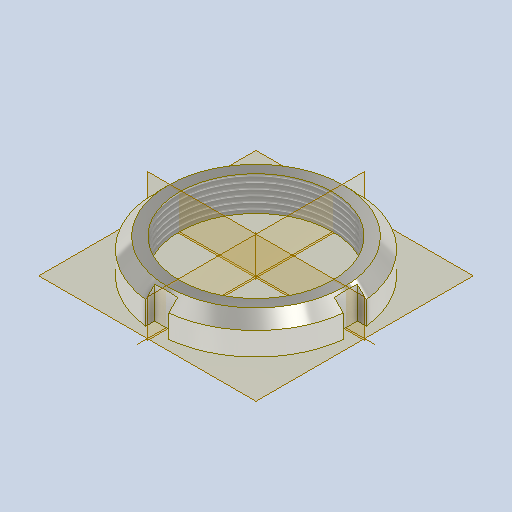
# Autodesk Inventor part: Sicherheitsmutter_m40
Saved by Autodesk Inventor 2022 (Build 260153000, 153)
## iProperties
Created: 2022-03-11
Part Number: Sicherheitsmutter_m40
Material: Generisch
Document SubType Name: Modeling
Designer: 123St
Density: 1 g/cm^3
Appearance: Silber
Mass: 6.67374 g
Surface Area: 40.864 cm^2
Volume: 6.67374 cm^3
Author: 123St
Autodesk Inventor part; units mm, degrees
sketch "Skizze1" plane through (0, 0, 0) normal (0, 1, 0) x (-1, 0, 0)
  circle A0 centre (0, 0) radius 20
  circle A1 centre (0, 0) radius 26
  dimension "d0" = 40
  dimension "d1" = 52
  constraints: 2 centre point, 2 coincident
  measures "d0" diameter of A0
  measures "d1" diameter of A1
extrude "Extrusion1" add sketch "Skizze1" along normal blind 9
chamfer "Fase1" distance 3 angle 45 1 edges at (26, 9, 0)
sketch "Skizze2" plane through (0, 9, 0) normal (0, 1, 0) x (1, 0, 0)
  line L0 (-28.5, -3) -> (-23.5, -3)
  line L1 (-23.5, -3) -> (-23.5, 3)
  line L2 (-23.5, 3) -> (-28.5, 3)
  line L3 (-28.5, 3) -> (-28.5, -3)
  circle A0 centre (0, 0) radius 26 projected
  line L4 (-28.5, -3) -> (-23.5, 3) construction
  line L5 (-23.5, -3) -> (-28.5, 3) construction
  line L6 (3, 23.5) -> (-3, 23.5)
  line L7 (-3, 23.5) -> (-3, 28.5)
  line L8 (-3, 28.5) -> (3, 28.5)
  line L9 (3, 28.5) -> (3, 23.5)
  line L10 (3, 23.5) -> (-3, 28.5) construction
  line L11 (-3, 23.5) -> (3, 28.5) construction
  line L12 (3, -23.5) -> (-3, -23.5)
  line L13 (-3, -23.5) -> (-3, -28.5)
  line L14 (-3, -28.5) -> (3, -28.5)
  line L15 (3, -28.5) -> (3, -23.5)
  line L16 (3, -23.5) -> (-3, -28.5) construction
  line L17 (-3, -23.5) -> (3, -28.5) construction
  line L18 (23.5, -3) -> (28.5, -3)
  line L19 (28.5, -3) -> (28.5, 3)
  line L20 (28.5, 3) -> (23.5, 3)
  line L21 (23.5, 3) -> (23.5, -3)
  line L22 (23.5, -3) -> (28.5, 3) construction
  line L23 (28.5, -3) -> (23.5, 3) construction
  line L24 (-39.9, 0) -> (39.9, 0) projected
  point P0 (-26, 0)
  point P1 (0, 26)
  point P2 (0, -26)
  point P3 (26, 0)
  dimension "d7" = 5
  dimension "d8" = 6
  dimension "d9" = 5
  dimension "d10" = 26
  dimension "d11" = 6
  dimension "d12" = 0
  dimension "d13" = 6
  dimension "d14" = 5
  dimension "d15" = 5
  dimension "d16" = 0
  constraints: 48 end point, 8 midpoint, 8 parallel, 4 horizontal, 4 perpendicular, 3 point on circle, 1 point on line
  measures "d7" distance of L6.end L7.end
  measures "d8" distance of L7.end L8.end
  measures "d9" distance of L19.end L20.end
  measures "d10" distance of A0.centre point (26, 0)
  measures "d11" distance of L18.end L19.end
  measures "d12" distance from line of L24 point (26, 0)
  measures "d13" distance of L13.end L14.end
  measures "d14" distance of L14.end L12.start
  measures "d15" distance of L1.end L2.end
  measures "d16" distance from line of L24 A0.start
extrude "Extrusion2" cut sketch "Skizze2" against normal blind 9 contours L3 L24 A0 L0 | A0 L24 L1 L0 | L3 L2 A0 L24 | A0 L2 L1 L24 | L13 L12 L15 A0 | A0 L15 L14 L13 | L24 A0 L18 L21 | L21 L20 A0 L24 | L7 L8 L9 A0 | A0 L9 L6 L7 | A0 L24 L19 L18 | A0 L20 L19 L24
thread "Gewinde1" size "M40x1.5" class "6H" standard "ANSI Metric M Profile" full length
